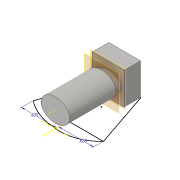
# Autodesk Inventor part: maleNT
Saved by Autodesk Inventor 2016 (Build 200138000, 138)
## iProperties
Created: 2016-01-27
Part Number: maleNT
Material: Generic
Document SubType Name: Modeling
Designer: 301278
Density: 1 g/cm^3
Appearance: Default
Author: 301278
Autodesk Inventor part; units mm, degrees
ref_plane "YZ Plane" through (0, 0, 0) normal (1, 0, 0) x (0, 1, 0)
ref_plane "XZ Plane" through (0, 0, 0) normal (0, 1, 0) x (-1, 0, 0)
ref_plane "XY Plane" through (0, 0, 0) normal (0, 0, 1) x (1, 0, 0)
sketch "Sketch1" plane through (0, 0, 0) normal (0, 0, 1) x (1, 0, 0)
  line L0 (0, 0) -> (14.605, 0)
  line L1 (14.605, 0) -> (14.605, 14.605)
  line L2 (14.605, 14.605) -> (0, 14.605)
  line L3 (0, 14.605) -> (0, 0)
  dimension "d0" = 14.605
  dimension "d1" = 14.605
  constraints: 8 end point, 2 parallel, 1 horizontal, 1 perpendicular
  measures "d0" distance of L2.end L1.end
  measures "d1" distance of L1.end L0.end
extrude "Extrusion1" add sketch "Sketch1" along normal blind 7.62
ref_plane "Work Plane1" through (0, 14.605, 7.62) normal (0, 0, 1) x (1, 0, 0)
sketch "Sketch2" plane through (0, 14.605, 7.62) normal (0, 0, 1) x (1, 0, 0)
  line L0 (14.605, 0) -> (0, 0) construction
  line L1 (0, 0) -> (7.3025, 0) construction
  line L2 (7.3025, 0) -> (14.605, 0) construction
  line L3 (7.3025, 0) -> (7.3025, -7.3025) construction
  ellipse E0 centre (7.3025, -7.3025) end of major axis (13.2969, -7.3025) minor radius 3.937
  point P0 (0, -14.605)
  dimension "d7" = 5.9944
  dimension "d8" = 3.937
  dimension "d4" = 7.3025
  dimension "d5" = 7.3025
  dimension "d6" = 7.3025
  constraints: 6 end point, 1 coincident, 1 collinear, 1 midpoint, 1 perpendicular, 2 other
  measures "d4" distance of L0.end L1.end
  measures "d5" distance of L1.end L0.start
  measures "d6" distance of L1.end L3.end
extrude "Extrusion2" add sketch "Sketch2" along normal blind 2.921
ref_plane "Work Plane2" through (0, 14.605, 10.541) normal (0, 0, 1) x (1, 0, 0)
sketch "Sketch3" plane through (0, 14.605, 10.541) normal (0, 0, 1) x (1, 0, 0)
  ellipse E0 centre (7.3025, -7.3076) end of major axis (13.8567, -7.3076) minor radius 5.2829
  ellipse E1 centre (7.3025, -7.3025) end of major axis (1.3081, -7.3025) minor radius 3.937 projected
  point P0 (0, -14.605)
  dimension "d12" = 0
  constraints: 3 other
  measures "d12" horizontal distance of point (7.302, -7.302) point (7.302, -7.308)
extrude "Extrusion3" add sketch "Sketch3" along normal blind 21.336 contours E0 | E1
sketch "Sketch4" plane through (0, 0, 0) normal (0, -1, 0) x (1, 0, 0)
  point P0 (0, 0)
sketch "Sketch5" plane through (0, 0, 0) normal (0, -1, 0) x (1, 0, 0)
  line L0 (7.3025, -6.3754) -> (7.3025, 38.2524) projected
  line L1 (14.605, 0) -> (0, 0) projected
  line L2 (14.605, 0) -> (23.4315, 25.9571)
  line L3 (0, 0) -> (-8.8368, 25.9535)
  line L4 (7.3025, 25.9553) -> (23.4315, 25.9571)
  line L5 (13.8567, 31.877) -> (0.7483, 31.877) projected
  arc A0 (7.3025, 31.877) -> (-8.8368, 25.9535) centre (8.5286, 3.5875) ccw
  arc A1 (23.4315, 25.9571) -> (7.3025, 31.877) centre (9.459, 12.8205) ccw
  dimension "d15" = 16.1393
  dimension "d16" = 16.129
  constraints: 6 end point, 4 point on circle, 2 centre point, 1 equal length, 1 midpoint, 1 point on line
  measures "d15" distance from line of L0 L3.end
  measures "d16" distance from line of L2.end L0
body "Solid1"
